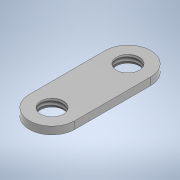
# Autodesk Inventor part: linkToActuator4
Saved by Autodesk Inventor 2021 (Build 250183000, 183)
## iProperties
Created: 2021-01-03
Part Number: linkToActuator4
Material: Generic
Document SubType Name: Modeling
Designer: awitc
Density: 1 g/cm^3
Appearance: Smooth - Medium Gray
Author: awitc
Autodesk Inventor part; units mm, degrees
ref_plane "YZ Plane" through (0, 0, 0) normal (1, 0, 0) x (0, 1, 0)
ref_plane "XZ Plane" through (0, 0, 0) normal (0, 1, 0) x (-1, 0, 0)
ref_plane "XY Plane" through (0, 0, 0) normal (0, 0, 1) x (1, 0, 0)
sketch "Sketch2" plane through (0, 0, 0) normal (0, 1, 0) x (-1, 0, 0)
  line L0 (0, 0) -> (6, 0)
  line L1 (6, 0) -> (0, 0)
  line L2 (0, -10) -> (6, -10)
  line L3 (3, 0) -> (8, 0)
  line L4 (8, -10) -> (3, -10)
  line L5 (3, -10) -> (-2, -10)
  line L6 (-2, 0) -> (3, 0)
  circle A0 centre (3, 0) radius 1.5
  circle A1 centre (3, 0) radius 3
  circle A2 centre (3, -10) radius 1.5
  circle A3 centre (3, -10) radius 3
  line L7 (0, 0) -> (0, -10)
  line L8 (6, 0) -> (6, -10)
  dimension "d24" = 10
  dimension "d30" = 5
  dimension "d31" = 5
  dimension "d32" = 3
  dimension "d33" = 6
  dimension "d34" = 3
  dimension "d35" = 6
  constraints: 18 end point, 4 centre point, 4 horizontal, 4 tangent, 3 parallel, 2 coincident, 1 point on line, 1 vertical
  measures "d24" distance of L2.start L1.end
  measures "d30" distance of L4.start L4.end
  measures "d31" distance of L6.start L6.end
  measures "d32" diameter of A0
  measures "d33" diameter of A1
  measures "d34" diameter of A2
  measures "d35" diameter of A3
extrude "Extrusion4" add sketch "Sketch2" along normal blind 1 contours A0 L0 A1 | L0 A1 A0 | L8 A3 L7 A1 | A3 L2 A2 | L2 A2 A3
thread "Thread1" size "M3x0.5" class "6H" standard "ANSI Metric M Profile" length 1
thread "Thread2" size "M3x0.5" class "6H" standard "ANSI Metric M Profile" length 1
body "Solid4"
